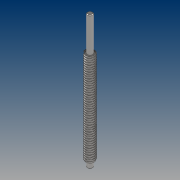
# Autodesk Inventor part: Truc_vit
Saved by Autodesk Inventor 2021 (Build 250183000, 183)
## iProperties
Created: 2024-04-08
Part Number: Truc_vit
Material: Stainless Steel, Austenitic
Document SubType Name: Modeling
Designer: Admin
Density: 8 g/cm^3
Appearance: Semi-Polished
Author: Admin
Autodesk Inventor part; units mm, degrees
ref_plane "YZ Plane" through (0, 0, 0) normal (1, 0, 0) x (0, 1, 0)
ref_plane "XZ Plane" through (0, 0, 0) normal (0, 1, 0) x (-1, 0, 0)
ref_plane "XY Plane" through (0, 0, 0) normal (0, 0, 1) x (1, 0, 0)
sketch "Sketch1" plane through (0, 0, 0) normal (1, 0, 0) x (0, 1, 0)
  line L0 (0, 0) -> (200, 0)
  line L1 (0, 0) -> (0, -4)
  line L2 (0, -4) -> (9, -4)
  line L3 (9, -4) -> (9, -6)
  line L4 (9, -6) -> (148, -6)
  line L5 (148, -6) -> (148, -4)
  line L6 (148, -4) -> (200, -4)
  line L7 (200, -4) -> (200, 0)
  dimension "d0" = 9
  dimension "d1" = 4
  dimension "d2" = 6
  dimension "d3" = 52
  dimension "d4" = 200
  constraints: 16 end point, 5 perpendicular, 2 point on line, 1 horizontal, 1 vertical
  measures "d0" distance between parallel lines of L1 L3
  measures "d1" distance between parallel lines of L0 L2
  measures "d2" distance between parallel lines of L0 L4
  measures "d3" distance between parallel lines of L5 L7
  measures "d4" distance between parallel lines of L1 L7
revolve "Revolution1" add sketch "Sketch1" angle 360 about axis through (0, 0, 0) along (0, 1, 0)
sketch "Sketch2" plane through (0, 0, 0) normal (1, 0, 0) x (0, 1, 0)
  line L0 (148, 6) -> (148, -6) projected
  line L1 (9, 6) -> (9, -6) projected
  line L2 (9, -6) -> (9.364, -7)
  line L3 (9.364, -7) -> (10.364, -7)
  line L4 (10.364, -7) -> (10.7279, -6)
  line L5 (148, -6) -> (9, -6) projected
  point P0 (0, 0)
  dimension "d6" = 1
  dimension "d7" = 70
  dimension "d8" = 1
  dimension "d9" = 139
  constraints: 6 end point, 1 equal length, 1 horizontal, 1 point on line
  measures "d6" distance of L2.end L3.end
  measures "d7" angle of L5 L4
  measures "d8" distance between parallel lines of L5 L3
  measures "d9" distance from line of L1.start L0
coil "Coil1" sketch "Sketch2" operation add axis through (0, -10, 0) along (0, 1, 0) pitch 3 turns 46.333333 hand right
chamfer "Chamfer1" distance 1 angle 45 2 edges at (0, 0, 4) (0, 200, 4)
equation "\"d11\" = d9"
body "Solid1"
